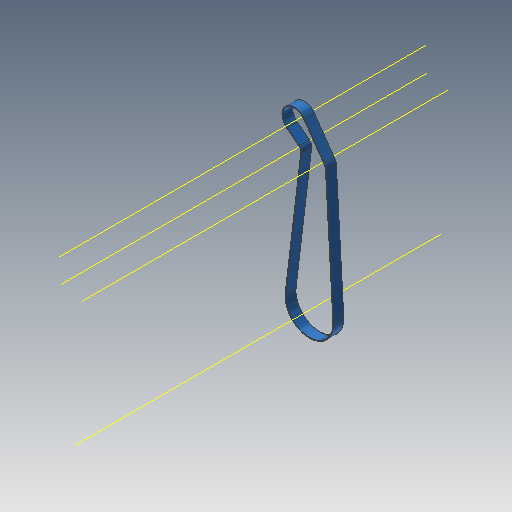
# Autodesk Inventor part: 歯付きベルト
Saved by Autodesk Inventor 2019.4 (Build 234330000, 330)
## iProperties
Created: 2019-11-13
Part Number: 歯付きベルト
Material: Rubber
Document SubType Name: Modeling
Designer: y6tada
Density: 1 g/cm^3
Appearance: シアン
CustomPartVersion: 1
Author: y6tada
Autodesk Inventor part; units mm, degrees
ref_plane "YZ Plane" through (0, 0, 0) normal (1, 0, 0) x (0, 1, 0)
ref_plane "XZ Plane" through (0, 0, 0) normal (0, 1, 0) x (-1, 0, 0)
ref_plane "XY Plane" through (0, 0, 0) normal (0, 0, 1) x (1, 0, 0)
sketch "スケッチ パス" plane through (0, 0, 0) normal (0, 0, 1) x (1, 0, 0)
  arc A0 (-17.312621, -71.176623) -> (20.715874, -72.352094) centre (1.649293, -73.457429) ccw
  arc A1 (-4.900605, 32.013061) -> (-6.547022, 35.93405) centre (-9.169832, 32.526579) ccw
  arc A2 (-2.585427, 56.430974) -> (-16.236335, 43.392143) centre (-10.411684, 50.959342) ccw
  arc A3 (14.799261, 29.707072) -> (13.518986, 33.396295) centre (7.649293, 29.292571) ccw
  line L0 (14.799261, 29.707072) -> (20.715874, -72.352094)
  line L1 (-17.312621, -71.176623) -> (-4.900605, 32.013061)
  line L2 (-6.547022, 35.93405) -> (-16.236335, 43.392143)
  line L3 (-2.585427, 56.430974) -> (13.518986, 33.396295)
  constraints: 8 end point, 8 point on circle, 4 centre point
ref_plane "断面平面" through (20.715874, -72.352094, 0) normal (-0.0578752, 0.9983238, 0) x (0, 0, 1)
ref_plane "作業平面2" through (1.649293, -73.457429, 0) normal (-1, 0, 0) x (0, 0, 1)
ref_plane "作業平面3" through (-10.411684, 50.959342, 0) normal (0.6399195, -0.768442, 0) x (0, 0, 1)
ref_plane "作業平面4" through (7.649293, 29.292571, 0) normal (-0.442179, 0.8969268, 0) x (0, 0, 1)
sketch "断面" plane through (20.715874, -72.352094, 0) normal (-0.0578752, 0.9983238, 0) x (0, 0, 1)
  line L0 (-4, 0.3) -> (4, 0.3)
  line L1 (4, 0.3) -> (4, -0.3)
  line L2 (4, -0.3) -> (-4, -0.3)
  line L3 (-4, -0.3) -> (-4, 0.3)
  line L4 (-4, 0) -> (4, 0) construction
  point P0 (0, 0)
  point P1 (0, 0)
  dimension "d0" = 8
  dimension "d4" = 0.3
  dimension "d5" = 0.3
  constraints: 10 end point, 3 midpoint, 2 parallel, 1 coincident, 1 horizontal, 1 perpendicular, 1 other
  measures "d0" distance between parallel lines of L1 L3
  measures "d4" distance between parallel lines of L2 L4
  measures "d5" distance between parallel lines of L4 L0
sweep "ベルト" add profiles "断面" path "スケッチ パス" path curves L3 A3 L0 A0 L1 A1 L2 A2
equation "\"d4\" = da_a"
equation "\"d5\" = da_a2"
equation "\"da_B\" = 6"
equation "\"da_pb\" = 2.5"
equation "\"da_L\" = 351.20212"
equation "\"da_a\" = 0.3"
equation "\"da_S\" = 1.5"
equation "\"da_Beta\" = 20deg"
equation "\"da_Ht\" = 0.7"
equation "\"da_H\" = 1.3"
equation "\"da_a2\" = 0.3"
body "Solid1"
